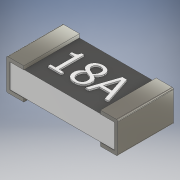
# Autodesk Inventor part: 21-1001
Saved by Autodesk Inventor 2018 (Build 220112000, 112)
## iProperties
Created: 2019-09-21
Part Number: 21-1001
Material: Copper
Document SubType Name: Modeling
Designer: Bradley
Density: 8.94 g/cm^3
Appearance: Smooth - White
Author: Bradley
Autodesk Inventor part; units mm, degrees
ref_plane "YZ Plane" through (0, 0, 0) normal (1, 0, 0) x (0, 1, 0)
ref_plane "XZ Plane" through (0, 0, 0) normal (0, 1, 0) x (-1, 0, 0)
ref_plane "XY Plane" through (0, 0, 0) normal (0, 0, 1) x (1, 0, 0)
sketch "Sketch1" plane through (0, 0, 0) normal (0, 1, 0) x (-1, 0, 0)
  line L0 (0.75, 0.175) -> (-0.75, 0.175)
  line L1 (-0.75, 0.175) -> (-0.75, -0.175)
  line L2 (-0.75, -0.175) -> (0.75, -0.175)
  line L3 (0.75, -0.175) -> (0.75, 0.175)
  line L4 (0.55, 0.175) -> (0.55, 0.225)
  line L5 (0.55, 0.225) -> (0.8, 0.225)
  line L6 (0.8, 0.225) -> (0.8, -0.225)
  line L7 (0.8, -0.225) -> (0.55, -0.225)
  line L8 (0.55, -0.225) -> (0.55, -0.175)
  line L9 (-0.55, 0.175) -> (-0.55, 0.225)
  line L10 (-0.55, 0.225) -> (-0.8, 0.225)
  line L11 (-0.8, 0.225) -> (-0.8, -0.225)
  line L12 (-0.8, -0.225) -> (-0.55, -0.225)
  line L13 (-0.55, -0.175) -> (-0.55, -0.225)
  line L14 (0.55, 0.175) -> (-0.55, 0.175)
  point P0 (0, 0)
  point P1 (0, 0.175)
  point P2 (0.75, 0)
  dimension "d0" = 1.6
  dimension "d1" = 0.05
  dimension "d2" = 0.05
  dimension "d3" = 0.45
  dimension "d4" = 0.25
  constraints: 30 end point, 12 point on line, 7 perpendicular, 3 collinear, 3 midpoint, 2 parallel, 1 horizontal, 1 horizontal alignment, 1 vertical, 1 vertical alignment
  measures "d0" distance between parallel lines of L11 L6
  measures "d1" distance of L7.end L8.end
  measures "d2" distance between parallel lines of L6 L3
  measures "d3" distance of L5.end L6.end
  measures "d4" distance of L6.end L7.end
extrude "Extrusion1" add sketch "Sketch1" along normal mid plane 0.8 contours L0 L4 L5 L6 L7 L8 L2 L3 | L0 L1 L2 L13 L12 L11 L10 L9
extrude "Extrusion2" add sketch "Sketch1" along normal mid plane 0.79 contours L3 L2 L1 L0
sketch "Sketch2" plane through (-0.55, -0.395, 0.175) normal (0, 0, 1) x (1, 0, 0)
  line L0 (0, 0) -> (0, 0.79) projected
  line L1 (1.1, 0) -> (0, 0) projected
  line L2 (1.1, 0) -> (1.1, 0.79) projected
  line L3 (0, 0.79) -> (1.1, 0.79) projected
  line L4 (0, 0.395) -> (1.1, 0.395) construction
  line L5 (0.338, 0.195) -> (0.1429, 0.195)
  line L6 (0.1429, 0.195) -> (0.1429, 0.2358)
  line L7 (0.1429, 0.2358) -> (0.2155, 0.2358)
  line L8 (0.2155, 0.2358) -> (0.2155, 0.5039)
  line L9 (0.2155, 0.5039) -> (0.1429, 0.5039)
  line L10 (0.1429, 0.5039) -> (0.1429, 0.5405)
  spline S0 degree 2 poles (0.1429, 0.5405) (0.184, 0.5405) (0.2229, 0.5639) (0.2255, 0.5963) knots 0 0 0 1 2 2 2
  line L11 (0.2255, 0.5963) -> (0.267, 0.5963)
  line L12 (0.267, 0.5963) -> (0.267, 0.2358)
  line L13 (0.267, 0.2358) -> (0.338, 0.2358)
  line L14 (0.338, 0.2358) -> (0.338, 0.195)
  spline S1 degree 2 poles (0.5325, 0.1859) (0.5027, 0.1859) (0.4537, 0.2038) (0.4365, 0.2203) knots 0 0 0 1 2 2 2
  spline S2 degree 2 poles (0.4365, 0.2203) (0.4197, 0.2365) (0.4022, 0.2806) (0.4022, 0.3055) knots 0 0 0 1 2 2 2
  spline S3 degree 2 poles (0.4022, 0.3055) (0.4022, 0.3379) (0.4369, 0.3924) (0.4699, 0.4086) knots 0 0 0 1 2 2 2
  line L15 (0.4699, 0.4086) -> (0.4699, 0.4102)
  spline S4 degree 2 poles (0.4699, 0.4102) (0.4404, 0.4274) (0.4119, 0.4683) (0.4119, 0.4987) knots 0 0 0 1 2 2 2
  spline S5 degree 2 poles (0.4119, 0.4987) (0.4119, 0.5438) (0.48, 0.6041) (0.5325, 0.6041) knots 0 0 0 1 2 2 2
  spline S6 degree 2 poles (0.5325, 0.6041) (0.587, 0.6041) (0.6528, 0.547) (0.6528, 0.5023) knots 0 0 0 1 2 2 2
  spline S7 degree 2 poles (0.6528, 0.5023) (0.6528, 0.4754) (0.6213, 0.4229) (0.5918, 0.408) knots 0 0 0 1 2 2 2
  line L16 (0.5918, 0.408) -> (0.5918, 0.4063)
  spline S8 degree 2 poles (0.5918, 0.4063) (0.6268, 0.3901) (0.6628, 0.3435) (0.6628, 0.3065) knots 0 0 0 1 2 2 2
  spline S9 degree 2 poles (0.6628, 0.3065) (0.6628, 0.2553) (0.5882, 0.1859) (0.5325, 0.1859) knots 0 0 0 1 2 2 2
  spline S10 degree 2 poles (0.6077, 0.3013) (0.6077, 0.326) (0.5882, 0.3551) (0.5607, 0.37) knots 0 0 0 1 2 2 2
  spline S11 degree 2 poles (0.5607, 0.37) (0.5516, 0.3752) (0.5212, 0.3872) (0.502, 0.395) knots 0 0 0 1 2 2 2
  spline S12 degree 2 poles (0.502, 0.395) (0.48, 0.3804) (0.4563, 0.337) (0.4563, 0.3094) knots 0 0 0 1 2 2 2
  spline S13 degree 2 poles (0.4563, 0.3094) (0.4563, 0.2731) (0.5001, 0.2258) (0.5331, 0.2258) knots 0 0 0 1 2 2 2
  spline S14 degree 2 poles (0.5331, 0.2258) (0.5669, 0.2258) (0.6077, 0.2663) (0.6077, 0.3013) knots 0 0 0 1 2 2 2
  spline S15 degree 2 poles (0.6002, 0.5016) (0.6002, 0.5285) (0.5643, 0.5645) (0.5322, 0.5645) knots 0 0 0 1 2 2 2
  spline S16 degree 2 poles (0.5322, 0.5645) (0.503, 0.5645) (0.4657, 0.5324) (0.4657, 0.5049) knots 0 0 0 1 2 2 2
  spline S17 degree 2 poles (0.4657, 0.5049) (0.4657, 0.4851) (0.4848, 0.4576) (0.504, 0.4465) knots 0 0 0 1 2 2 2
  spline S18 degree 2 poles (0.504, 0.4465) (0.5121, 0.442) (0.5464, 0.4261) (0.5604, 0.4216) knots 0 0 0 1 2 2 2
  spline S19 degree 2 poles (0.5604, 0.4216) (0.5837, 0.4394) (0.6002, 0.4773) (0.6002, 0.5016) knots 0 0 0 1 2 2 2
  line L17 (0.68, 0.195) -> (0.8148, 0.595)
  line L18 (0.8148, 0.595) -> (0.8803, 0.595)
  line L19 (0.8803, 0.595) -> (1.0152, 0.195)
  line L20 (1.0152, 0.195) -> (0.9591, 0.195)
  line L21 (0.9591, 0.195) -> (0.9228, 0.3068)
  line L22 (0.9228, 0.3068) -> (0.7701, 0.3068)
  line L23 (0.7701, 0.3068) -> (0.7338, 0.195)
  line L24 (0.7338, 0.195) -> (0.68, 0.195)
  line L25 (0.9082, 0.3522) -> (0.8463, 0.5405)
  line L26 (0.8463, 0.5405) -> (0.7847, 0.3522)
  line L27 (0.7847, 0.3522) -> (0.9082, 0.3522)
  point P0 (0.55, 0.395)
  constraints: 2 end point, 2 midpoint, 1 horizontal
extrude "Extrusion3" add sketch "Sketch2" along normal blind 0.02 contours L5 L6 L7 L8 L9 L10 S0 L11 L12 L13 L14 | S1 S2 S3 S4 S5 S6 S7 S8 S9 | L17 L18 L19 L20 L21 L22 L23 L24
fillet "Fillet1" radius 0.02 4 edges at (-0.8, 0, 0.225) (-0.8, 0, -0.225) (0.8, 0, 0.225) (0.8, 0, -0.225)
equation "\"d2\" = d1"
body "Solid1"
